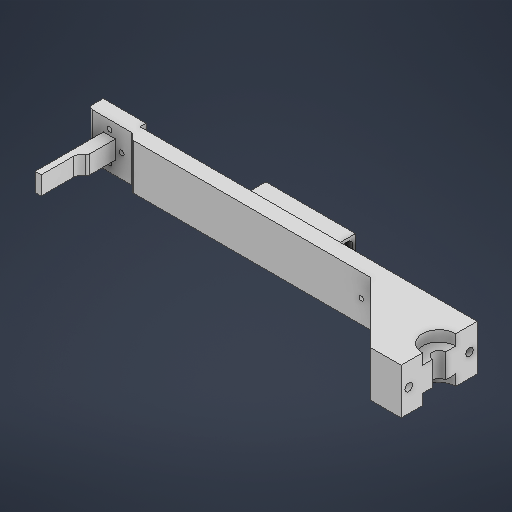
# Autodesk Inventor part: PeçaCerta
Saved by Autodesk Inventor 2026 (Build 300175050, 175E)
## iProperties
Created: 2025-03-07
Part Number: PeçaCerta
Material: Genérico
Document SubType Name: Modeling
Designer: Ian
Density: 1 g/cm^3
Appearance: Padrão
Mass: 116.041 g
Surface Area: 272.444 cm^2
Volume: 116.041 cm^3
Author: Ian
Autodesk Inventor part; units mm, degrees
ref_plane "YZ Plane" through (0, 0, 0) normal (1, 0, 0) x (0, 1, 0)
ref_plane "XZ Plane" through (0, 0, 0) normal (0, 1, 0) x (-1, 0, 0)
ref_plane "XY Plane" through (0, 0, 0) normal (0, 0, 1) x (1, 0, 0)
sketch "Esboço1" plane through (0, 0, 0) normal (0, 0, 1) x (1, 0, 0)
  circle A0 centre (-0.0013, -9.4999) radius 1.5997
  circle A1 centre (8, 0) radius 1.6001
  circle A2 centre (-8, 0) radius 1.5997
  circle A3 centre (0, 0) radius 3
  circle A4 centre (-0.0004, 9.5) radius 1.6001
  line L0 (0, 9.8096) -> (0, -11.1096)
  line L1 (-6.3022, 0) -> (16.3218, 0)
  line L2 (-14.0997, 15) -> (235.9003, 15)
  line L3 (235.9003, 15) -> (235.9003, -15)
  line L4 (235.9003, -15) -> (-14.0997, -15)
  line L5 (-14.0997, -15) -> (-14.0997, 15)
  point P0 (-14.0997, 0)
  dimension "d13" = 18.9999
  dimension "d37" = 9.2196
  dimension "d38" = 9.2197
  dimension "d39" = 9.2198
  dimension "d42" = 6.0001
  dimension "d43" = 16
  dimension "d45" = 9.2207
  dimension "d46" = 4.5
  dimension "d47" = 250
  dimension "d48" = 30
  dimension "d49" = 0
  constraints: 12 end point, 5 centre point, 3 horizontal, 2 equal radius, 2 point on line, 2 vertical, 1 coincident, 1 midpoint, 1 parallel, 1 perpendicular
  measures "d13" distance of A4.centre A0.centre
  measures "d42" diameter of A3
  measures "d43" distance of A1.centre A2.centre
  measures "d46" distance edge to line of A2 L5
  measures "d47" distance of L2.start L2.end
  measures "d48" distance of L4.end L2.start
  measures "d49" vertical distance of A3.centre point (-14.1, 0)
extrude "Extrusão7" add sketch "Esboço1" along normal blind 10
sketch "Esboço10" plane through (0, 0, 0) normal (0, 0, -1) x (-1, 0, 0)
  circle A0 centre (-8, 0) radius 1.6001 projected
  line L0 (-145.9003, 15) -> (-86.9003, 15)
  line L1 (-86.9003, 15) -> (-86.9003, -15)
  line L2 (-86.9003, -15) -> (-145.9003, -15)
  line L3 (-145.9003, -15) -> (-145.9003, 15)
  line L4 (-145.9003, 15) -> (-86.9003, -15) construction
  line L5 (-86.9003, 15) -> (-145.9003, -15) construction
  line L6 (-145.9003, 13.5) -> (-86.9003, 13.5)
  line L7 (-86.9003, -13.5) -> (-145.9003, -13.5)
  line L8 (-235.9003, -15) -> (-235.9003, 15) projected
  point P0 (0, 0)
  point P1 (-116.4003, 0)
  dimension "d135" = 59
  dimension "d136" = 30
  dimension "d180" = 1.5
  dimension "d181" = 1.5
  dimension "d182" = 90
  constraints: 16 end point, 4 point on line, 3 horizontal, 3 parallel, 2 midpoint, 1 perpendicular
  measures "d135" distance of L1.end L2.end
  measures "d136" distance of L0.end L1.end
  measures "d180" distance between parallel lines of L2 L7
  measures "d181" distance between parallel lines of L0 L6
  measures "d182" distance between parallel lines of L8 L3
extrude "Extrusão8" add sketch "Esboço10" along normal blind 10 contours L0 L1 L6 L3 | L6 L1 L7 L3 | L7 L1 L2 L3
sketch "Esboço13" plane through (0, 0, 0) normal (0, 0, -1) x (-1, 0, 0)
  line L0 (14.0997, -15) -> (-235.9003, -15) projected
  circle A0 centre (8, 0) radius 1.5997 projected
  circle A1 centre (0, 0) radius 3 projected
  circle A2 centre (0.0013, -9.4999) radius 1.5997 projected
  circle A3 centre (-8, 0) radius 1.6001 projected
  circle A4 centre (0.0004, 9.5) radius 1.6001 projected
  circle A5 centre (0, 0) radius 3
  circle A6 centre (-8, 0) radius 1.6001
  circle A7 centre (0.0013, -9.4999) radius 1.5997
  circle A8 centre (8, 0) radius 1.5997
  circle A9 centre (0.0004, 9.5) radius 1.6001
  line L1 (14.0997, 15) -> (14.0997, -15) projected
  line L2 (-14.0997, 15) -> (14.0997, 15)
  line L3 (14.0997, 15) -> (14.0997, -15)
  line L4 (14.0997, -15) -> (-14.0997, -15)
  line L5 (-14.0997, -15) -> (-14.0997, 15)
  line L6 (-14.0997, 15) -> (14.0997, -15) construction
  line L7 (14.0997, 15) -> (-14.0997, -15) construction
  point P0 (0, 0)
  point P1 (-15, -15)
  point P2 (-14.0997, -15)
  constraints: 12 end point, 5 centre point, 5 coincident, 5 concentric, 2 midpoint, 2 parallel, 1 horizontal, 1 perpendicular, 1 point on line
extrude "Extrusão11" add sketch "Esboço13" along normal blind 4
sketch "Esboço14" plane through (0, 0, 10) normal (0, 0, 1) x (1, 0, 0)
  line L0 (235.9003, 15) -> (-14.0997, 15) projected
  line L1 (14.0997, -15) -> (-14.0997, -15)
  line L2 (-14.0997, -15) -> (-14.0997, 15)
  line L3 (-14.0997, 15) -> (14.0997, 15)
  line L4 (14.0997, 15) -> (14.0997, -15)
  line L5 (14.0997, -15) -> (-14.0997, 15) construction
  line L6 (-14.0997, -15) -> (14.0997, 15) construction
  line L7 (14.0997, -15) -> (19.0997, -15)
  line L8 (19.0997, -15) -> (19.0997, 15)
  line L9 (19.0997, 15) -> (14.0997, 15)
  line L10 (14.0997, 15) -> (14.0997, -15)
  point P0 (0, 0)
  dimension "d240" = 5
  constraints: 20 end point, 4 parallel, 2 horizontal, 2 midpoint, 2 perpendicular, 1 point on line
  measures "d240" distance of L9.end L8.end
extrude "Extrusão12" cut sketch "Esboço14" against normal blind 4
sketch "Esboço15" plane through (235.9003, 15, 10) normal (0, 1, 0) x (1, 0, 0)
  line L0 (0, 0) -> (-216.8006, 0) projected
  line L1 (-216.8006, 0) -> (-220.8006, 4)
  line L2 (-220.8006, 4) -> (-216.8006, 4)
  line L3 (-216.8006, 4) -> (-216.8006, 0) projected
  line L4 (-216.8006, 0) -> (-216.8006, 4)
  point P0 (-235.9003, 10)
  dimension "d241" = 135
  constraints: 6 end point, 1 horizontal, 1 vertical
  measures "d241" angle of L0 L1
extrude "Extrusão13" add sketch "Esboço15" against normal up to surface (30 mm away)
fillet "Arredondamento4" radius 1 2 edges at (19.0997, 0, 10) (15.0997, 0, 6)
fillet "Arredondamento5" radius 3 1 edges at (-14.0997, 0, 6)
sketch "Esboço18" plane through (0, 0, 10) normal (0, 0, 1) x (1, 0, 0)
  line L0 (14.0997, -15) -> (235.9003, -15) projected
  line L1 (235.9003, 15) -> (14.0997, 15) projected
  line L2 (235.9003, -15) -> (175.9003, -15)
  line L3 (175.9003, -15) -> (175.9003, 15)
  line L4 (175.9003, 15) -> (235.9003, 15)
  line L5 (235.9003, 15) -> (235.9003, -15)
  point P0 (0, 0)
  dimension "d81" = 60
  constraints: 8 end point, 2 parallel, 1 horizontal, 1 perpendicular, 1 point on line
  measures "d81" distance of L3.end L4.end
extrude "Extrusão14" add sketch "Esboço18" along normal blind 40
sketch "Esboço19" plane through (14.0997, -15, 0) normal (0, -1, 0) x (1, 0, 0)
  line L0 (5.4142, 10) -> (161.8006, 10) projected
  line L1 (161.8006, 10) -> (201.8006, 50)
  line L2 (221.8006, 50) -> (161.8006, 50) projected
  line L3 (201.8006, 50) -> (161.8006, 50)
  line L4 (161.8006, 10) -> (161.8006, 50)
  point P0 (-14.0997, 0)
  point P1 (0.4142, 10)
  point P2 (10, 10)
  point P3 (5, 10)
  dimension "d84" = 45
  constraints: 6 end point, 1 collinear, 1 perpendicular, 1 point on line
  measures "d84" angle of L2 L1
extrude "Extrusão15" cut sketch "Esboço19" against normal through all
sketch "Esboço20" plane through (14.0997, -15, 0) normal (0, -1, 0) x (1, 0, 0)
  line L0 (161.8006, 10) -> (221.8006, 10)
  line L1 (221.8006, 0) -> (221.8006, 50) projected
  line L2 (221.8006, 50) -> (201.8006, 50) projected
  line L3 (201.8006, 50) -> (191.8006, 10)
  circle A0 centre (221.8006, 25) radius 10.975
  point P0 (-14.0997, 0)
  point P1 (221.8006, 35.975)
  point P2 (221.8006, 14.025)
  dimension "d87" = 21.95
  constraints: 4 end point, 2 midpoint, 1 centre point, 1 horizontal, 1 point on line
  measures "d87" diameter of A0
extrude "Extrusão16" cut sketch "Esboço20" against normal blind 7 contours A0 L1 picked at (218.1689, 24.559)
sketch "Esboço21" plane through (14.0997, -8, 0) normal (0, -1, 0) x (1, 0, 0)
  line L0 (221.8006, 35.975) -> (221.8006, 14.025) projected
  arc A0 (221.8006, 35.975) -> (221.8006, 14.025) centre (221.8006, 25) ccw projected
  circle A1 centre (221.8006, 25) radius 4.25
  point P0 (-14.0997, 0)
  point P1 (221.8006, 20.75)
  point P2 (221.8006, 29.25)
  dimension "d90" = 8.5
  constraints: 1 centre point, 1 coincident
  measures "d90" diameter of A1
extrude "Extrusão17" cut sketch "Esboço21" against normal through all contours L0 A1 picked at (220.3943, 24.8292)
sketch "Esboço22" plane through (14.0997, 15, 0) normal (0, 1, 0) x (1, 0, 0)
  arc A0 (221.8006, -20.75) -> (221.8006, -29.25) centre (221.8006, -25) ccw projected
  circle A1 centre (221.8006, -25) radius 10.975
  point P0 (-14.0997, 0)
  dimension "d93" = 21.95
  dimension "d173" = 4.25
  constraints: 1 centre point, 1 coincident
  measures "d93" diameter of A1
  measures "d173" radius of A0
extrude "Extrusão18" cut sketch "Esboço22" against normal blind 7
sketch "Esboço23" plane through (235.9003, -15, 0) normal (1, 0, 0) x (0, 0, -1)
  line L0 (-14.025, 30) -> (-14.025, 23) projected
  line L1 (-14.025, 7) -> (-14.025, 0) projected
  line L2 (-10, 0) -> (-10, 30) projected
  line L3 (-10, 30) -> (0, 30)
  circle A0 centre (-5, 15) radius 2.5
  line L4 (0, 15) -> (-50, 15)
  line L5 (-50, 30) -> (-50, 0) projected
  line L6 (-20.75, 23) -> (-20.75, 7) projected
  circle A1 centre (-45, 15) radius 2.5
  line L7 (-29.25, 7) -> (-29.25, 23) projected
  dimension "d96" = 5
  dimension "d174" = 15.75
  dimension "d175" = 5
  dimension "d177" = 15.75
  constraints: 4 end point, 2 centre point, 1 horizontal, 1 midpoint, 1 point on line
  measures "d96" diameter of A0
  measures "d174" distance from line of L6 A0.centre
  measures "d175" diameter of A1
  measures "d177" distance from line of L7 A1.centre
extrude "Extrusão19" cut sketch "Esboço23" against normal blind 50
sketch "Esboço24" plane through (0, 0, 0) normal (0, 0, -1) x (-1, 0, 0)
  line L0 (-235.9003, -2.5) -> (-235.9003, 2.5) projected
  line L1 (-175.9003, -15) -> (-175.9003, 15) projected
  line L2 (-183.4003, -12.5) -> (-208.4003, -12.5)
  line L3 (-208.4003, -12.5) -> (-208.4003, 12.5)
  line L4 (-208.4003, 12.5) -> (-183.4003, 12.5)
  line L5 (-183.4003, 12.5) -> (-183.4003, -12.5)
  line L6 (-183.4003, -12.5) -> (-208.4003, 12.5) construction
  line L7 (-208.4003, -12.5) -> (-183.4003, 12.5) construction
  point P0 (0, 0)
  dimension "d101" = 25
  dimension "d102" = 25
  constraints: 12 end point, 2 parallel, 1 horizontal, 1 perpendicular
  measures "d101" distance of L3.end L4.end
  measures "d102" distance of L2.end L3.end
extrude "Extrusão20" cut sketch "Esboço24" against normal through all
sketch "Esboço33" plane through (0, 0, 0) normal (0, 0, -1) x (-1, 0, 0)
  line L0 (-235.9003, -15) -> (-235.9003, 15) projected
  circle A0 centre (-169.6038, 0) radius 1.5
  point P0 (0, 0)
  dimension "d121" = 3
  dimension "d122" = 66.2965
  constraints: 1 centre point, 1 coincident
  measures "d121" diameter of A0
  measures "d122" distance from line of A0.centre L0
extrude "Extrusão25" cut sketch "Esboço33" against normal blind 10
sketch "Esboço35" plane through (145.9003, -15, 0) normal (1, 0, 0) x (0, 0, -1)
  line L0 (10, 30) -> (10, 0) projected
  line L1 (8, 28) -> (0, 28)
  line L2 (0, 28) -> (0, 2)
  line L3 (0, 2) -> (8, 2)
  line L4 (8, 2) -> (8, 28)
  line L5 (0, 30) -> (10, 30) projected
  line L6 (0, 30) -> (0, 0)
  line L7 (-0.0048, 28.7972) -> (-0.0048, 0.7972)
  point P0 (0, 15)
  point P1 (0, 30)
  dimension "d13" = 18.9999
  dimension "d37" = 9.2196
  dimension "d38" = 9.2197
  dimension "d39" = 9.2198
  dimension "d42" = 6.0001
  dimension "d43" = 16
  dimension "d45" = 9.2207
  dimension "d46" = 4.5
  dimension "d47" = 250
  dimension "d48" = 30
  dimension "d49" = 0
  dimension "d139" = 8
  dimension "d140" = 26
  dimension "d141" = 0
  dimension "d142" = 2
  constraints: 12 end point, 2 parallel, 1 horizontal, 1 perpendicular, 1 vertical
  measures "d139" distance of L3.end L2.end
  measures "d140" distance of L2.end L1.end
  measures "d141" distance between parallel lines of L6 L2
  measures "d142" distance between parallel lines of L5 L1
extrude "Extrusão26" cut sketch "Esboço35" against normal up to surface (59 mm away)
sketch "Esboço38" plane through (0, 0, 6) normal (0, 0, 1) x (1, 0, 0)
  line L0 (-4, -6) -> (4, -6)
  line L1 (4, -6) -> (4, 6)
  line L2 (4, 6) -> (-4, 6)
  line L3 (-4, 6) -> (-4, -6)
  line L4 (-4, -6) -> (4, 6) construction
  line L5 (4, -6) -> (-4, 6) construction
  point P0 (0, 0)
  dimension "d154" = 8
  dimension "d155" = 12
  constraints: 12 end point, 2 midpoint, 2 parallel, 1 horizontal, 1 perpendicular
  measures "d154" distance of L2.end L1.end
  measures "d155" distance of L1.end L0.end
extrude "Extrusão29" add sketch "Esboço38" along normal blind 45
sketch "Esboço39" plane through (-4, 6, 6) normal (0, 1, 0) x (1, 0, 0)
  line L0 (8, -45) -> (4, -45)
  line L1 (4, -45) -> (4, -23.875)
  line L2 (4, -23.875) -> (8, -23.875)
  line L3 (8, -23.875) -> (8, -45)
  line L4 (8, 0) -> (8, -45) projected
  arc A0 (8, -18.3181) -> (4, -23.875) centre (9.8599, -23.875) ccw
  line L5 (8, -18.3181) -> (8, -23.875)
  point P0 (4, 6)
  dimension "d158" = 4
  dimension "d159" = 21.125
  constraints: 10 end point, 2 parallel, 2 point on circle, 1 centre point, 1 collinear, 1 horizontal, 1 perpendicular, 1 point on line, 1 tangent
  measures "d158" distance of L1.end L2.end
  measures "d159" distance of L0.end L1.end
extrude "Extrusão30" cut sketch "Esboço39" against normal through all
fillet "Arredondamento6" radius 2 1 edges at (4, 0, 24.3181)
sketch "Esboço42" plane through (0, 0, 50) normal (0, 0, 1) x (1, 0, 0)
  line L0 (208.4003, 12.5) -> (208.4003, 0) projected
  line L1 (208.4003, 0) -> (208.4003, -12.5) projected
  line L2 (215.9003, 15) -> (215.9003, -15) projected
  line L3 (208.4003, 12.5) -> (215.9003, 12.5)
  line L4 (215.9003, 12.5) -> (215.9003, -12.5)
  line L5 (215.9003, -12.5) -> (208.4003, -12.5)
  line L6 (208.4003, -12.5) -> (208.4003, 12.5)
  point P0 (0, 0)
  constraints: 8 end point, 2 parallel, 1 horizontal, 1 perpendicular, 1 point on line
extrude "Extrusão33" cut sketch "Esboço42" against normal blind 10
sketch "Esboço43" plane through (0, 0, -10) normal (0, 0, -1) x (-1, 0, 0)
  line L0 (-86.9003, -15) -> (-86.9003, 15) projected
  line L1 (-145.9003, -15) -> (-86.9003, -15) projected
  line L2 (-145.9003, 15) -> (-145.9003, -15) projected
  line L3 (-86.9003, 15) -> (-145.9003, 15) projected
  line L4 (-145.9003, 13) -> (-86.9003, 13) projected
  line L5 (-145.9003, -13) -> (-86.9003, -13) projected
  line L6 (-86.9003, 13) -> (-145.9003, 13)
  line L7 (-145.9003, 13) -> (-145.9003, -13)
  line L8 (-145.9003, -13) -> (-86.9003, -13)
  line L9 (-86.9003, -13) -> (-86.9003, 13)
  line L10 (-91.9003, 13) -> (-91.9003, -13)
  line L11 (-140.9003, 13) -> (-140.9003, -13)
  point P0 (0, 0)
  point P1 (-140.9003, 13)
  point P2 (-140.9003, -13)
  point P3 (-91.9003, 13)
  dimension "d233" = 5
  dimension "d234" = 5
  constraints: 12 end point, 4 point on line, 3 perpendicular, 2 parallel, 1 horizontal
  measures "d233" distance between parallel lines of L0 L10
  measures "d234" distance between parallel lines of L2 L11
extrude "Extrusão34" cut sketch "Esboço43" against normal up to surface (10 mm away) contours L5 L11 L4 L10
chamfer "Chanfro1" distance 7.5 angle 45 1 edges at (208.4003, 0, 40)
chamfer "Chanfro2" distance 2 angle 45 4 edges at (143.4003, -13, -8) (143.4003, 13, -8) (89.4003, -13, -8) (89.4003, 13, -8)
fillet "Arredondamento7" radius 5 1 edges at (183.4003, 0, 0)
sketch "Esboço44" plane through (183.4003, -12.5, 17.5) normal (1, 0, 0) x (0, 0, -1)
  point P0 (17.5, 12.5)
sketch "Esboço45" plane through (183.4003, -12.5, 17.5) normal (1, 0, 0) x (0, 0, -1)
  line L0 (12.5, 25) -> (0, 25) projected
  line L1 (12.5, 0) -> (0, 0) projected
  line L2 (12.5, 25) -> (0, 25)
  line L3 (0, 25) -> (0, 0)
  line L4 (0, 0) -> (12.5, 0)
  line L5 (12.5, 0) -> (12.5, 25)
  line L6 (10.5, 25) -> (2, 25)
  line L7 (2, 25) -> (2, 0)
  line L8 (2, 0) -> (10.5, 0)
  line L9 (10.5, 0) -> (10.5, 25)
  line L10 (10.5, 23) -> (2, 23)
  line L11 (10.5, 2) -> (2, 2)
  point P0 (17.5, 12.5)
  dimension "d246" = 2
  dimension "d247" = 2
  dimension "d248" = 2
  dimension "d249" = 2
  constraints: 20 end point, 6 point on line, 4 parallel, 4 perpendicular, 2 horizontal
  measures "d246" distance between parallel lines of L5 L9
  measures "d247" distance between parallel lines of L3 L7
  measures "d248" distance between parallel lines of L1 L11
  measures "d249" distance between parallel lines of L10 L0
extrude "Extrusão35" add sketch "Esboço45" along normal blind 5 contours L9 L11 L7 L10
sketch "Esboço46" plane through (183.4003, -10.5, 7) normal (0, 0, -1) x (-1, 0, 0)
  line L0 (0, -2) -> (0, 23) projected
  line L1 (0, 19) -> (-3, 19)
  line L2 (-3, 19) -> (-3, 2)
  line L3 (-3, 2) -> (0, 2)
  line L4 (0, 2) -> (0, 19)
  line L5 (0, 0) -> (-5, 0) projected
  line L6 (-5, 0) -> (-5, 21) projected
  line L7 (0, 21) -> (-5, 21) projected
  point P0 (183.4003, 10.5)
  point P1 (-2.5, 21)
  point P2 (0, 2)
  dimension "d252" = 2
  dimension "d253" = 2
  dimension "d254" = 2
  constraints: 8 end point, 2 parallel, 1 horizontal, 1 midpoint, 1 perpendicular, 1 point on line
  measures "d252" distance between parallel lines of L5 L3
  measures "d253" distance between parallel lines of L6 L2
  measures "d254" distance from line of point (-2.5, 21) L1
extrude "Extrusão36" cut sketch "Esboço46" against normal blind 10 contours L3 L2 L1 L0
fillet "Arredondamento8" radius 2 2 edges at (188.4003, 10.5, 11.25) (188.4003, -10.5, 11.25)
